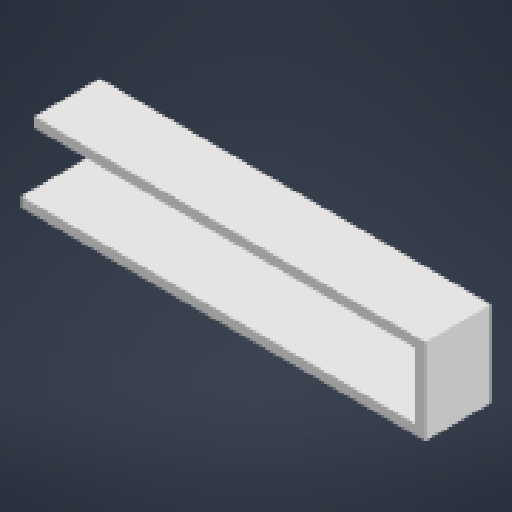
# Autodesk Inventor part: enclosure__bone_bottom_left
Saved by Autodesk Inventor 2026.2 (Build 302298000, 298)
## iProperties
Created: 2026-04-20
Part Number: enclosure__bone_bottom_left
Material: Generic
Document SubType Name: Modeling
Designer: Alvin
Density: 1 g/cm^3
Appearance: Default
Author: Alvin
Autodesk Inventor part; units mm, degrees
sketch "Sketch1" plane through (0, 0, 0) normal (0, 1, 0) x (-1, 0, 0)
  line L0 (58.5, 10) -> (-58.5, 10)
  line L1 (-58.5, 10) -> (-58.5, -10)
  line L2 (-58.5, -10) -> (58.5, -10)
  line L3 (58.5, -10) -> (58.5, 10)
  line L4 (58.5, 10) -> (-58.5, -10) construction
  line L5 (-58.5, 10) -> (58.5, -10) construction
  point P0 (0, 0)
  dimension "d0" = 20
  dimension "d1" = 117
  constraints: 12 end point, 2 midpoint, 2 parallel, 1 horizontal, 1 perpendicular
  measures "d0" distance of L2.end L0.start
  measures "d1" distance of L0.start L0.end
extrude "Extrusion1" add sketch "Sketch1" along normal blind 3
sketch "Sketch2" plane through (58.5, 0, 10) normal (1, 0, 0) x (0, 0, -1)
  line L0 (20, 0) -> (20, 3) projected
  line L1 (0, 3) -> (20, 3) projected
  line L2 (0, 0) -> (0, 3) projected
  line L3 (150, -20) -> (0, -20) projected
  line L4 (20, 0) -> (20, -20)
  line L5 (0, 0) -> (0, -20)
  line L6 (20, -20) -> (20, -23)
  line L7 (20, -23) -> (0, -23)
  line L8 (0, -23) -> (0, -20)
  point P0 (10, 0)
  dimension "d4" = 3
  constraints: 10 end point, 3 perpendicular, 1 parallel, 1 point on line, 1 vertical
  measures "d4" distance of L4.end L6.end
extrude "Extrusion2" add sketch "Sketch2" along normal blind 3
sketch "Sketch3" plane through (58.5, -23, -10) normal (0, -1, 0) x (1, 0, 0)
  line L0 (0, 20) -> (0, 0) projected
  line L1 (-121, 20) -> (-121, -3) projected
  line L2 (0, 0) -> (-121, 0)
  line L3 (0, 20) -> (-121, 20)
  point P0 (-58.5, 10)
  constraints: 4 end point, 1 parallel, 1 perpendicular, 1 point on line
ref_plane "Work Plane1" through (-251.5, -20, -8.5) normal (0, -1, 0) x (1, 0, 0)
extrude "Extrusion3" add sketch "Sketch3" against normal up to surface (3 mm away)
sketch "Sketch4" plane through (-62.5, -23, -10) normal (-1, 0, 0) x (0, 0, 1)
  line L0 (0, 3) -> (20, 3) projected
  line L1 (0, 0) -> (0, 3) projected
  line L2 (20, 0) -> (0, 0) projected
  line L3 (20, 0) -> (20, 3) projected
  point P0 (10, 23)
ref_plane "Work Plane2" through (-61.5, -23, -10) normal (1, 0, 0) x (0, 1, 0)
extrude "Extrusion4" cut sketch "Sketch4" against normal up to surface (1 mm away)
sketch "Sketch5" plane through (-58.5, 0, -10) normal (-1, 0, 0) x (0, 0, 1)
  line L0 (0, 0) -> (20, 0) projected
  line L1 (20, 0) -> (20, 3) projected
  line L2 (0, 3) -> (20, 3) projected
  line L3 (0, 0) -> (0, 3) projected
  point P0 (10, 0)
ref_plane "Work Plane3" through (-57.5, 4, -10) normal (1, 0, 0) x (0, 1, 0)
extrude "Extrusion5" cut sketch "Sketch5" against normal up to surface (1 mm away)
sketch "Sketch6" plane through (58.5, -23, 10) normal (0, 0, 1) x (1, 0, 0)
  line L0 (-116, 26) -> (-116, 23) projected
  line L1 (-116, 23) -> (0, 23) projected
  line L2 (0, 23) -> (0, 3) projected
  line L3 (0, 3) -> (0, 0) projected
  line L4 (0, 0) -> (3, 0) projected
  line L5 (3, 26) -> (3, 0) projected
  line L6 (-116, 26) -> (3, 26) projected
  line L7 (-1.5, 3) -> (-1.5, 3) projected
  line L8 (-2.3, 7.5) -> (-2.3, 7.5) projected
  line L9 (-2.3, 7.5) -> (-2.3, 7.5) projected
  line L10 (-120, 3) -> (-120, 0) projected
  line L11 (0, 0) -> (-120, 0) projected
  line L12 (0, 3) -> (0, 0) projected
  line L13 (-120, 3) -> (0, 3) projected
  line L14 (-20, 16.6) -> (-20, 21.5) projected
  line L15 (-116, 26) -> (3, 26) projected
  line L16 (-20, 26) -> (-20, 21.5)
  line L17 (-20, 16.6) -> (-20, 0)
  line L18 (-20, 0) -> (-20, 1.5)
  point P0 (-58.5, 23)
  point P1 (-20, 3)
  point P2 (-20, 23)
  constraints: 6 end point, 4 point on line, 1 perpendicular
ref_plane "Work Plane4" through (-274.5, -23, 75) normal (0, 0, 1) x (1, 0, 0)
extrude "Extrusion6" add sketch "Sketch6" along normal up to surface (65 mm away) contours L6 L5 L4 L3 L2 L1 L16 | L3 L11 L17 L13
sketch "Sketch7" plane through (61.5, -23, 75) normal (1, 0, 0) x (0, 0, -1)
  circle A0 centre (-23.75, 13) radius 2 projected
  circle A1 centre (18.75, 13) radius 2 projected
  point P0 (75, 23)
ref_plane "Work Plane5" through (58.5, -6.4, -10) normal (1, 0, 0) x (0, 1, 0)
extrude "Extrusion7" cut sketch "Sketch7" against normal up to surface (3 mm away)
sketch "Sketch8" plane through (-61.5, -23, -10) normal (0, -1, 0) x (1, 0, 0)
  line L0 (0, 20) -> (0, 0) projected
  line L1 (0, 0) -> (123, 0) projected
  line L2 (123, 20) -> (123, 0) projected
  line L3 (123, 20) -> (123, 85) projected
  line L4 (123, 85) -> (100, 85) projected
  line L5 (100, 20) -> (100, 85) projected
  line L6 (100, 20) -> (0, 20) projected
  line L7 (0, 10) -> (123, 10) construction
  circle A0 centre (30.75, 10) radius 2
  circle A1 centre (92.25, 10) radius 2
  point P0 (61.5, 10)
  dimension "d17" = 4
  dimension "d18" = 4
  dimension "d19" = 30.75
  dimension "d20" = 30.75
  constraints: 2 centre point, 2 end point, 2 midpoint, 2 point on line
  measures "d17" diameter of A0
  measures "d18" diameter of A1
  measures "d19" distance from line of L0 A0.centre
  measures "d20" distance from line of L2 A1.centre
extrude "Extrusion8" cut sketch "Sketch8" against normal up to surface (26 mm away) contours A0 | A1
fillet "Fillet1" radius 5 4 edges at (61.5, -23, 0) (61.5, -23, 42.5) (61.5, 3, 0) (61.5, 3, 42.5)
move faces "Move1" translate (0, 0, 65) faces at (59.5, -12.6667, 75)
sketch "Sketch9" plane through (61.5, -18, 10) normal (1, 0, 0) x (0, 0, -1)
  circle A0 centre (-46.25, 8) radius 2 projected
  point P0 (10, 18)
extrude "Extrusion9" add sketch "Sketch9" against normal blind 3
sketch "Sketch10" plane through (61.5, -18, 10) normal (1, 0, 0) x (0, 0, -1)
  circle A0 centre (-88.75, 8) radius 2 projected
  circle A1 centre (-46.25, 8) radius 2 projected
  point P0 (10, 18)
extrude "Extrusion10" cut sketch "Sketch10" against normal blind 3
sketch "Sketch11" plane through (38.5, 0, 140) normal (0, 0, 1) x (1, 0, 0)
  arc A0 (23, -2) -> (18, 3) centre (18, -2) ccw projected
  line L0 (0, 3) -> (18, 3) projected
  line L1 (0, 0) -> (0, 3) projected
  line L2 (20, 0) -> (0, 0) projected
  line L3 (20, -20) -> (20, 0) projected
  line L4 (0, -20) -> (20, -20) projected
  line L5 (0, -23) -> (0, -20) projected
  line L6 (18, -23) -> (0, -23) projected
  arc A1 (18, -23) -> (23, -18) centre (18, -18) ccw projected
  line L7 (23, -2) -> (23, -18) projected
  line L8 (20, -20) -> (20, -20) projected
  line L9 (20, -20) -> (20, -13.4174)
  line L10 (20, 0) -> (20, 2.5826)
  point P0 (-38.5, 0)
  constraints: 4 end point, 2 point on circle, 1 perpendicular, 1 point on line
ref_plane "Work Plane6" through (-271.5, -18.5, 160) normal (0, 0, 1) x (1, 0, 0)
extrude "Extrusion11" add sketch "Sketch11" along normal up to surface (20 mm away) contours L7 A1 L6 L5 L4 L3 L10 A0
body "Solid1"
